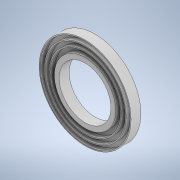
# Autodesk Inventor part: labyrinth
Saved by Autodesk Inventor 2021 (Build 250183000, 183)
## iProperties
Created: 2020-12-28
Part Number: labyrinth
Material: Generic
Document SubType Name: Modeling
Designer: Angelos
Density: 1 g/cm^3
Appearance: Default
Author: Angelos
Autodesk Inventor part; units mm, degrees
ref_plane "YZ Plane" through (0, 0, 0) normal (1, 0, 0) x (0, 1, 0)
ref_plane "XZ Plane" through (0, 0, 0) normal (0, 1, 0) x (-1, 0, 0)
sketch "Sketch1" plane through (0, 0, 0) normal (0, 0, 1) x (1, 0, 0)
  circle A0 centre (0, 0) radius 71.5
  circle A1 centre (0, 0) radius 73.5
  circle A2 centre (0, 0) radius 81.5
  circle A3 centre (0, 0) radius 83.5
  circle A4 centre (0, 0) radius 91.5
  circle A5 centre (0, 0) radius 93.5
  circle A6 centre (0, 0) radius 52.5
  circle A7 centre (0, 0) radius 62.5
  dimension "d0" = 143
  dimension "d1" = 147
  dimension "d2" = 163
  dimension "d3" = 167
  dimension "d4" = 183
  dimension "d5" = 187
  dimension "d6" = 105
  dimension "d7" = 125
  constraints: 8 centre point, 8 coincident
  measures "d0" diameter of A0
  measures "d1" diameter of A1
  measures "d2" diameter of A2
  measures "d3" diameter of A3
  measures "d4" diameter of A4
  measures "d5" diameter of A5
  measures "d6" diameter of A6
  measures "d7" diameter of A7
extrude "Extrusion1" add sketch "Sketch1" along normal blind 10
extrude "Extrusion2" add sketch "Sketch1" against normal blind 10 contours A0 | A1 | A2 | A3 | A4 | A5 | A6 | A7
extrude "Extrusion3" cut sketch "Sketch1" against normal blind 10 contours A6
ref_plane "Work Plane4" through (0, 0, -5) normal (0, 0, 1) x (1, 0, 0)
ref_plane "Work Plane3" through (0, 0, 0) normal (0, 0, 1) x (1, 0, 0)
sketch "Sketch3" plane through (0, 0, 10) normal (0, 0, 1) x (1, 0, 0)
  circle A0 centre (0, 0) radius 61
  dimension "d18" = 122
  constraints: 1 centre point, 1 coincident
  measures "d18" diameter of A0
sketch "Sketch4" plane through (0, 0, 5) normal (0, 0, 1) x (1, 0, 0)
  circle A0 centre (0, 0) radius 61
  dimension "d19" = 122
  constraints: 1 centre point, 1 coincident
  measures "d19" diameter of A0
sketch "Sketch5" plane through (0, 0, 0) normal (0, 0, 1) x (1, 0, 0)
  circle A0 centre (0, 0) radius 61
  dimension "d20" = 122
  constraints: 1 centre point, 1 coincident
  measures "d20" diameter of A0
ref_plane "Work Plane1" through (0, 0, 10) normal (0, 0, 1) x (1, 0, 0)
ref_plane "Work Plane2" through (0, 0, 5) normal (0, 0, 1) x (1, 0, 0)
body "Solid1"
